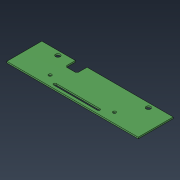
# Autodesk Inventor part: Ballsensorplatine
Saved by Autodesk Inventor 2022.3 (Build 263350000, 350)
## iProperties
Part Number: Ballsensorplatine
Material: Phenolharz
Document SubType Name: Modeling
Designer: rYan
Density: 1.38 g/cm^3
Appearance: Glatt - waldgrün
Mass: 3.47544 g
Surface Area: 54.0002 cm^2
Volume: 2.51843 cm^3
Author: rYan
Autodesk Inventor part; units mm, degrees
ref_plane "YZ Plane" through (0, 0, 0) normal (1, 0, 0) x (0, 1, 0)
ref_plane "XZ Plane" through (0, 0, 0) normal (0, 1, 0) x (-1, 0, 0)
ref_plane "XY Plane" through (0, 0, 0) normal (0, 0, 1) x (1, 0, 0)
sketch "Skizze1" plane through (0, 0, 0) normal (0, 0, 1) x (1, 0, 0)
  line L0 (-45, 12) -> (45, 12)
  line L1 (45, 12) -> (45, -12)
  line L2 (45, -12) -> (-45, -12)
  line L3 (-45, -12) -> (-45, 12)
  line L4 (-45, 12) -> (45, -12) construction
  line L5 (45, 12) -> (-45, -12) construction
  point P0 (0, 0)
  dimension "d0" = 24
  dimension "d1" = 90
  constraints: 12 end point, 2 midpoint, 2 parallel, 1 horizontal, 1 perpendicular
  measures "d0" distance of L0.end L1.end
  measures "d1" distance of L0.start L0.end
extrude "Extrusion1" add sketch "Skizze1" along normal blind 1
sketch "Skizze4" plane through (0, 0, 1) normal (0, 0, 1) x (1, 0, 0)
  line L0 (15, -9.1) -> (-15, -9.1) construction
  line L1 (15, -8.2) -> (-15, -8.2)
  line L2 (-15, -10) -> (15, -10)
  arc A0 (15, -10) -> (15, -8.2) centre (15, -9.1) ccw
  arc A1 (-15, -8.2) -> (-15, -10) centre (-15, -9.1) ccw
  line L3 (0, 17) -> (0, -18) projected
  line L4 (-45, -12) -> (45, -12) projected
  point P0 (0, 0)
  point P1 (0, -9.1)
  dimension "d25" = 1.8
  dimension "d26" = 30
  dimension "d27" = 2
  constraints: 8 end point, 4 point on circle, 4 tangent, 2 centre point, 1 horizontal, 1 midpoint, 1 parallel, 1 other
  measures "d25" diameter of A1
  measures "d26" distance of L0.start L0.end
  measures "d27" distance between parallel lines of L4 L2
extrude "Extrusion2" cut sketch "Skizze4" against normal through all
sketch "Skizze2" plane through (0, 0, 1) normal (0, 0, 1) x (1, 0, 0)
  line L0 (31, 9) -> (-31, 9) construction
  line L1 (45, 12) -> (-45, 12) projected
  line L2 (0, 20.4) -> (0, -17.4) projected
  line L3 (-45, -12) -> (45, -12) projected
  dimension "d5" = 62
  dimension "d48" = 21
  constraints: 2 coincident, 2 end point, 1 symmetric about line
  measures "d5" distance of L0.start L0.end
  measures "d48" distance between parallel lines of L0 L3
hole "Bohrung1" at (-31, 9, 1) at (31, 9, 1) direction (0, 0, -1) diameter 3.1 end through all
sketch "Skizze5" plane through (0, 0, 1) normal (0, 0, 1) x (1, 0, 0)
  line L0 (-45, -12) -> (45, -12) projected
  line L1 (0, 17.4) -> (0, -20.4) projected
  point P0 (0, 0)
  point P1 (22.05, -5.3)
  point P2 (-22.05, -5.3)
  dimension "d30" = 6.7
  dimension "d31" = 44.1
  constraints: 1 symmetric about line
  measures "d30" distance from line of L0 point (22.05, -5.3)
  measures "d31" distance of point (-22.05, -5.3) point (22.05, -5.3)
hole "Bohrung3" at (22.05, -5.3, 1) at (-22.05, -5.3, 1) direction (0, 0, -1) diameter 2.1 end through all
sketch "Skizze7" plane through (0, 0, 1) normal (0, 0, 1) x (1, 0, 0)
  line L0 (0, 20.4) -> (0, -17.4) projected
  line L1 (-45, -12) -> (45, -12) projected
  line L2 (-22, 12) -> (-14, 12)
  line L3 (-14, 12) -> (-14, 5)
  line L4 (-14, 5) -> (-22, 5)
  line L5 (-22, 5) -> (-22, 12)
  line L6 (-18, 5) -> (-18, 12) construction
  line L7 (45, 12) -> (-45, 12) construction
  point P0 (0, 0)
  dimension "d49" = 18
  dimension "d50" = 17
  dimension "d51" = 8
  constraints: 10 end point, 2 midpoint, 2 parallel, 1 collinear, 1 horizontal, 1 perpendicular
  measures "d49" distance between parallel lines of L0 L6
  measures "d50" distance between parallel lines of L1 L4
  measures "d51" distance between parallel lines of L3 L5
extrude "Extrusion4" cut sketch "Skizze7" against normal through all
chamfer "Fase1" distance 1 angle 45 2 edges at (-22, 5, 0.5) (-14, 5, 0.5)
